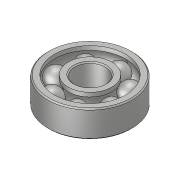
# Autodesk Inventor part: bearing
Saved by Autodesk Inventor 2017 (Build 210142000, 142)
## iProperties
Created: 2017-06-09
Part Number: bearing
Material: Stainless Steel AISI 304
Document SubType Name: Modeling
Designer: Tobias
Density: 8 g/cm^3
Appearance: Chrome - Satin
Mass: 10.806 g
Surface Area: 21.8227 cm^2
Volume: 1.35075 cm^3
Author: Tobias
Autodesk Inventor part; units mm, degrees
ref_plane "YZ Plane" through (0, 0, 0) normal (1, 0, 0) x (0, 1, 0)
ref_plane "XZ Plane" through (0, 0, 0) normal (0, 1, 0) x (-1, 0, 0)
ref_plane "XY Plane" through (0, 0, 0) normal (0, 0, 1) x (1, 0, 0)
sketch "Sketch2" plane through (0, 0, 0) normal (1, 0, 0) x (0, 1, 0)
  line L0 (0, 4.9) -> (0, -4.9) projected
  line L1 (11, 3.5) -> (9.3, 3.5)
  line L2 (9.3, -3.5) -> (11, -3.5)
  line L3 (11, -3.5) -> (11, 3.5)
  line L4 (5.7, 3.5) -> (4, 3.5)
  line L5 (4, 3.5) -> (4, -3.5)
  line L6 (4, -3.5) -> (5.7, -3.5)
  line L7 (-2.2, 0) -> (13.2, 0) projected
  line L8 (9.3, 3.5) -> (9.3, 2.4289)
  line L9 (9.3, -2.4289) -> (9.3, -3.5)
  line L10 (5.7, -3.5) -> (5.7, -2.4289)
  line L11 (5.7, 2.4289) -> (5.7, 3.5)
  ellipse E0 centre (7.5, 0) end of major axis (7.5, -3.5) minor radius 2.5 (9.3, -2.4289) -> (9.3, 2.4289) ccw
  ellipse E1 centre (7.5, 0) end of major axis (7.5, -3.5) minor radius 2.5 (5.7, 2.4289) -> (5.7, -2.4289) ccw
  point P0 (0, 0)
  point P1 (9.3, 2.0819)
  point P2 (5.7, 2.0819)
  dimension "d7" = 4
  dimension "d8" = 11
  dimension "d9" = 7
  dimension "d18" = 1.7
  dimension "d19" = 1.7
  dimension "d24" = 1.7
  dimension "d25" = 1.7
  constraints: 20 end point, 6 parallel, 5 point on line, 3 perpendicular, 2 horizontal, 9 other
  measures "d7" distance between parallel lines of L0 L5
  measures "d8" distance between parallel lines of L0 L3
  measures "d9" distance between parallel lines of L2 L1
  measures "d18" distance between parallel lines of L5 L11
  measures "d19" distance between parallel lines of L8 L3
  measures "d24" distance between parallel lines of L9 L3
  measures "d25" distance between parallel lines of L5 L10
revolve "Revolution1" add sketch "Sketch2" angle 360 about axis through (0, 0, 0) along (0, 0, -1)
chamfer "Chamfer2" distance 0.3 angle 45 4 edges at (0, -11, 3.5) (0, -11, -3.5) (0, -4, 3.5) (0, -4, -3.5)
sketch "Sketch3" plane through (0, 0, 0) normal (1, 0, 0) x (0, 1, 0)
  line L0 (-15.4, 0) -> (15.4, 0) projected
  arc A0 (7.5, -2.5) -> (7.5, 2.5) centre (7.5, 0) ccw
  line L1 (-9.3, -2.4289) -> (9.3, -2.4289) projected
  line L2 (7.5, 2.5) -> (7.5, -2.5)
  point P0 (0, 0)
  dimension "d29" = 7.5
  dimension "d30" = 5
  constraints: 2 end point, 2 point on circle, 1 centre point, 1 point on line
  measures "d29" distance of point (0, 0) A0.centre
  measures "d30" diameter of A0
revolve "Revolution2" add sketch "Sketch3" angle 360 about axis through (0, 7.5, 2.5) along (0, 0, -1)
pattern_circular "Circular Pattern1" count 7 over 360 about axis through (0, 0, -10) along (0, 0, 1) of "Revolution2"
body "Solid2"
